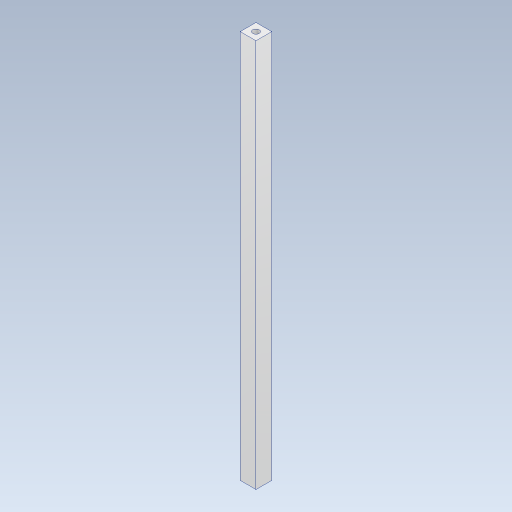
# Autodesk Inventor part: shaft
Saved by Autodesk Inventor 2024 (Build 280153000, 153)
## iProperties
Created: 2024-11-10
Part Number: shaft
Material: Aluminum 6061
Document SubType Name: Modeling
Designer: Oscar
Density: 2.7 g/cm^3
Appearance: Aluminum - Flat
Author: Oscar
Autodesk Inventor part; units mm, degrees
ref_plane "YZ Plane" through (0, 0, 0) normal (1, 0, 0) x (0, 1, 0)
ref_plane "XZ Plane" through (0, 0, 0) normal (0, 1, 0) x (-1, 0, 0)
ref_plane "XY Plane" through (0, 0, 0) normal (0, 0, 1) x (1, 0, 0)
sketch "Sketch1" plane through (0, 0, 0) normal (0, 1, 0) x (-1, 0, 0)
  line L0 (0, 0) -> (3.175, 0)
  line L1 (3.175, 0) -> (3.175, -3.175)
  line L2 (3.175, -3.175) -> (0, -3.175)
  line L3 (0, -3.175) -> (0, 0)
  point P0 (0, -1.5875)
  point P1 (3.175, -1.5875)
  dimension "d2" = 3.175
  dimension "d3" = 3.175
  constraints: 8 end point, 2 midpoint, 2 parallel, 1 horizontal, 1 perpendicular
  measures "d2" distance of L2.end L0.start
  measures "d3" distance of point (0, -1.587) point (3.175, -1.587)
extrude "Extrusion1" add sketch "Sketch1" along normal blind 78.1304
sketch "Sketch2" plane through (0, 78.1304, 0) normal (0, 1, 0) x (1, 0, 0)
  circle A0 centre (-1.5875, 1.5875) radius 0.635
  line L0 (0, 3.175) -> (-3.175, 3.175) construction
  line L1 (-3.175, 3.175) -> (0, 0) construction
  line L2 (-3.175, 3.175) -> (-3.175, 0) construction
  line L3 (0, 3.175) -> (-3.175, 0) construction
  dimension "d4" = 1.27
  constraints: 4 end point, 1 centre point, 1 coincident, 1 midpoint
  measures "d4" diameter of A0
extrude "Extrusion2" cut sketch "Sketch2" against normal blind 25.4
body "Solid1"
